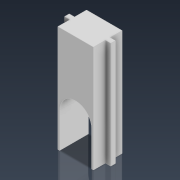
# Autodesk Inventor part: Slider-4
Saved by Autodesk Inventor 2021.1 (Build 251245010, 245A)
## iProperties
Created: 2020-12-20
Part Number: Slider-4
Material: 一般
Document SubType Name: Modeling
Designer: User
Density: 1 g/cm^3
Appearance: 預設
Author: User
Autodesk Inventor part; units mm, degrees
ref_plane "YZ Plane" through (0, 0, 0) normal (1, 0, 0) x (0, 1, 0)
ref_plane "XZ Plane" through (0, 0, 0) normal (0, 1, 0) x (-1, 0, 0)
ref_plane "XY Plane" through (0, 0, 0) normal (0, 0, 1) x (1, 0, 0)
sketch "草圖1" plane through (0, 0, 0) normal (0, 1, 0) x (-1, 0, 0)
  line L0 (-33.5, 27) -> (33.5, 27)
  line L1 (33.5, 27) -> (33.5, -27)
  line L2 (33.5, -27) -> (-33.5, -27)
  line L3 (-33.5, -27) -> (-33.5, 27)
  line L4 (-33.5, 27) -> (33.5, -27) construction
  line L5 (33.5, 27) -> (-33.5, -27) construction
  line L6 (43.5, -4.5) -> (33.5, -4.5)
  line L7 (33.5, -4.5) -> (33.5, 4.5)
  line L8 (33.5, 4.5) -> (43.5, 4.5)
  line L9 (43.5, 4.5) -> (43.5, -4.5)
  line L10 (-33.5, -4.5) -> (-43.5, -4.5)
  line L11 (-43.5, -4.5) -> (-43.5, 4.5)
  line L12 (-43.5, 4.5) -> (-33.5, 4.5)
  line L13 (-33.5, 4.5) -> (-33.5, -4.5)
  point P0 (0, 0)
  point P1 (33.5, 0)
  point P2 (-33.5, 0)
  point P3 (-33.5, 4.5)
  point P4 (-33.5, -4.5)
  dimension "d0" = 67
  dimension "d1" = 54
  dimension "d2" = 9
  dimension "d3" = 10
  constraints: 28 end point, 6 midpoint, 6 parallel, 3 horizontal, 3 perpendicular, 2 equal length
  measures "d0" distance of L0.start L0.end
  measures "d1" distance of L2.end L0.start
  measures "d2" distance of L8.end L6.start
  measures "d3" distance of L6.start L6.end
extrude "擠出1" add sketch "草圖1" along normal blind 250
sketch "草圖2" plane through (-33.5, 0, 27) normal (0, 0, 1) x (1, 0, 0)
  circle A0 centre (33.5, 102) radius 30
  line L0 (0, 0) -> (67, 0) projected
  line L1 (3.5, 102) -> (63.5, 102)
  line L2 (63.5, 102) -> (63.5, -30.9469)
  line L3 (63.5, -30.9469) -> (3.5, -30.9469)
  line L4 (3.5, -30.9469) -> (3.5, 102)
  point P0 (33.5, 0)
  point P1 (33.5, 0)
  point P2 (63.5, 102)
  dimension "d6" = 102
  dimension "d7" = 60
  constraints: 8 end point, 2 midpoint, 2 parallel, 1 centre point, 1 coincident, 1 horizontal, 1 perpendicular, 1 tangent, 1 vertical alignment
  measures "d6" distance from line of A0.centre L0
  measures "d7" diameter of A0
extrude "擠出2" cut sketch "草圖2" against normal through all
sketch "草圖3" plane through (-33.5, 250, 27) normal (0, 0, 1) x (1, 0, 0)
  line L0 (-69.9684, -200) -> (136.9684, -200)
  line L1 (136.9684, -200) -> (136.9684, -250)
  line L2 (136.9684, -250) -> (-69.9684, -250)
  line L3 (-69.9684, -250) -> (-69.9684, -200)
  point P0 (33.5, -250)
  point P1 (33.5, -250)
  dimension "d10" = 50
  constraints: 8 end point, 2 parallel, 1 coincident, 1 horizontal, 1 midpoint, 1 perpendicular
  measures "d10" distance of L0.end L1.end
extrude "擠出3" cut sketch "草圖3" against normal through all
sketch "草圖4" plane through (33.5, 250, -27) normal (0, 0, -1) x (-1, 0, 0)
  arc A0 (63.5, -148) -> (3.5, -148) centre (33.5, -148) ccw construction
  circle A1 centre (33.5, -136) radius 30
  line L0 (63.5, -200) -> (3.5, -200)
  line L1 (3.5, -200) -> (3.5, -136)
  line L2 (3.5, -136) -> (63.5, -136)
  line L3 (63.5, -136) -> (63.5, -200)
  point P0 (33.5, -250)
  point P1 (63.5, -200)
  dimension "d13" = 12
  dimension "d14" = 60
  constraints: 8 end point, 2 coincident, 2 parallel, 1 centre point, 1 horizontal, 1 midpoint, 1 perpendicular, 1 tangent, 1 vertical alignment
  measures "d13" distance of A0.centre A1.centre
  measures "d14" diameter of A1
sketch "草圖5" plane through (-33.5, 250, 27) normal (0, 0, 1) x (1, 0, 0)
  circle A0 centre (33.5, -134) radius 30
  arc A1 (63.5, -148) -> (3.5, -148) centre (33.5, -148) ccw construction
  line L0 (63.5, -200) -> (3.5, -200)
  line L1 (3.5, -200) -> (3.5, -134)
  line L2 (3.5, -134) -> (63.5, -134)
  line L3 (63.5, -134) -> (63.5, -200)
  point P0 (33.5, -250)
  dimension "d15" = 14
  dimension "d16" = 60
  constraints: 8 end point, 2 coincident, 2 parallel, 1 centre point, 1 horizontal, 1 midpoint, 1 perpendicular, 1 tangent, 1 vertical alignment
  measures "d15" distance of A1.centre A0.centre
  measures "d16" diameter of A0
loft "斷面混成1" cut profiles "草圖4", "草圖5"
